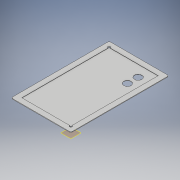
# Autodesk Inventor part: Lid
Saved by Autodesk Inventor 2019 (Build 230136000, 136)
## iProperties
Created: 2018-10-23
Part Number: Lid
Material: Generic
Document SubType Name: Modeling
Designer: Administrator
Density: 1 g/cm^3
Appearance: Default
Author: Administrator
Autodesk Inventor part; units mm, degrees
ref_plane "YZ Plane" through (0, 0, 0) normal (1, 0, 0) x (0, 1, 0)
ref_plane "XZ Plane" through (0, 0, 0) normal (0, 1, 0) x (-1, 0, 0)
ref_plane "XY Plane" through (0, 0, 0) normal (0, 0, 1) x (1, 0, 0)
ref_plane "Work Plane1" through (0, 41.656, 0) normal (0, 1, 0) x (1, 0, 0)
sketch "Sketch2" plane through (0, 41.656, 0) normal (0, 1, 0) x (1, 0, 0)
  line L0 (-118.364, 207.264) -> (-10.414, 207.264) projected
  arc A0 (-4.064, 200.914) -> (-10.414, 207.264) centre (-10.414, 200.914) ccw projected
  line L1 (-4.064, 200.914) -> (-4.064, 10.414) projected
  arc A1 (-10.414, 4.064) -> (-4.064, 10.414) centre (-10.414, 10.414) ccw projected
  line L2 (-10.414, 4.064) -> (-118.364, 4.064) projected
  arc A2 (-124.714, 10.414) -> (-118.364, 4.064) centre (-118.364, 10.414) ccw projected
  line L3 (-124.714, 10.414) -> (-124.714, 200.914) projected
  arc A3 (-118.364, 207.264) -> (-124.714, 200.914) centre (-118.364, 200.914) ccw projected
  line L4 (-128.778, 208.153) -> (-128.778, 3.175) projected
  arc A4 (-128.778, 3.175) -> (-125.603, 0) centre (-125.603, 3.175) ccw projected
  line L5 (-125.603, 0) -> (-3.175, 0) projected
  arc A5 (-3.175, 0) -> (0, 3.175) centre (-3.175, 3.175) ccw projected
  line L6 (0, 3.175) -> (0, 208.153) projected
  arc A6 (0, 208.153) -> (-3.175, 211.328) centre (-3.175, 208.153) ccw projected
  line L7 (-3.175, 211.328) -> (-125.603, 211.328) projected
  arc A7 (-125.603, 211.328) -> (-128.778, 208.153) centre (-125.603, 208.153) ccw projected
  circle A8 centre (-117.348, 199.898) radius 2.794 projected
  circle A9 centre (-11.43, 11.43) radius 2.794 projected
  line L8 (-117.348, 199.898) -> (-11.43, 199.898)
  line L9 (-11.43, 199.898) -> (-11.43, 11.43)
  line L10 (-11.43, 11.43) -> (-117.348, 11.43)
  line L11 (-117.348, 11.43) -> (-117.348, 199.898)
  point P0 (0, 0)
  constraints: 8 end point, 2 parallel, 1 horizontal, 1 perpendicular
extrude "Extrusion5" add sketch "Sketch2" along normal blind 1.27 contours L0 A0 L1 A1 L2 A2 L3 A3 | A7 L7 A6 L6 A5 L5 A4 L4
extrude "Extrusion6" add sketch "Sketch2" along normal blind 0.508 contours L8 L9 A9 L10 L11 A8 | A8 L11 L8 | L9 L10 A9 picked at (-115.5087, 199.6908) picked at (-13.2693, 11.6372)
sketch "Sketch3" plane through (0, 42.164, 0) normal (0, 1, 0) x (1, 0, 0)
  line L0 (-14.224, 11.43) -> (-117.348, 11.43) projected
  line L1 (-114.554, 199.898) -> (-11.43, 199.898) projected
  line L2 (-117.348, 11.43) -> (-62.992, 11.43)
  line L3 (-62.992, 11.43) -> (-62.992, 199.898)
  line L4 (-62.992, 199.898) -> (-117.348, 199.898)
  line L5 (-117.348, 199.898) -> (-117.348, 11.43)
  line L6 (-11.43, 199.898) -> (-62.992, 199.898)
  line L7 (-62.992, 199.898) -> (-62.992, 105.664)
  line L8 (-62.992, 105.664) -> (-11.43, 105.664)
  line L9 (-11.43, 105.664) -> (-11.43, 199.898)
  line L10 (-37.211, 105.664) -> (-62.992, 105.664)
  line L11 (-62.992, 105.664) -> (-62.992, 199.898)
  line L12 (-62.992, 199.898) -> (-37.211, 199.898)
  line L13 (-37.211, 199.898) -> (-37.211, 105.664)
  line L14 (-11.43, 199.898) -> (-11.43, 14.224) projected
  line L15 (-11.43, 199.898) -> (-37.211, 199.898)
  line L16 (-37.211, 199.898) -> (-37.211, 152.781)
  line L17 (-37.211, 152.781) -> (-11.43, 152.781)
  line L18 (-11.43, 152.781) -> (-11.43, 199.898)
  line L19 (-11.43, 105.664) -> (-24.3205, 105.664)
  line L20 (-24.3205, 105.664) -> (-24.3205, 199.898)
  line L21 (-24.3205, 199.898) -> (-11.43, 199.898)
  line L22 (-11.43, 199.898) -> (-11.43, 105.664)
  line L23 (-37.211, 176.3395) -> (-24.3205, 176.3395)
  line L24 (-24.3205, 176.3395) -> (-24.3205, 152.781)
  line L25 (-24.3205, 152.781) -> (-37.211, 152.781)
  line L26 (-37.211, 152.781) -> (-37.211, 176.3395)
  line L27 (-37.211, 105.664) -> (-24.3205, 105.664)
  line L28 (-24.3205, 105.664) -> (-24.3205, 152.781)
  line L29 (-24.3205, 152.781) -> (-37.211, 152.781)
  line L30 (-37.211, 152.781) -> (-37.211, 105.664)
  line L31 (-37.211, 129.2225) -> (-24.3205, 129.2225)
  line L32 (-24.3205, 129.2225) -> (-24.3205, 152.781)
  line L33 (-24.3205, 152.781) -> (-37.211, 152.781)
  line L34 (-37.211, 152.781) -> (-37.211, 129.2225)
  line L35 (-24.3205, 105.664) -> (-30.7657, 105.664)
  line L36 (-30.7657, 105.664) -> (-30.7657, 129.2225)
  line L37 (-30.7657, 129.2225) -> (-24.3205, 129.2225)
  line L38 (-24.3205, 129.2225) -> (-24.3205, 105.664)
  line L39 (-30.7657, 129.2225) -> (-24.3205, 129.2225)
  line L40 (-24.3205, 129.2225) -> (-24.3205, 199.898)
  line L41 (-24.3205, 199.898) -> (-30.7657, 199.898)
  line L42 (-30.7657, 199.898) -> (-30.7657, 129.2225)
  point P0 (0, 0)
  constraints: 80 end point, 20 parallel, 10 horizontal, 10 perpendicular, 9 midpoint
sketch "Sketch4" plane through (0, 42.164, 0) normal (0, 1, 0) x (1, 0, 0)
  point P0 (0, 0)
  point P1 (-30.9206, 152.9754)
  point P2 (-30.9206, 176.1357)
hole "Hole1" at (-30.9206, 42.164, -152.9754) at (-30.9206, 42.164, -176.1357) direction (0, -1, 0) diameter 16.002 depth 8.001 tip angle 118
sketch "Sketch5" plane through (0, 42.164, 0) normal (0, 1, 0) x (1, 0, 0)
  circle A0 centre (-30.9206, 152.9754) radius 8.001 projected
  circle A1 centre (-30.9206, 176.1357) radius 8.001 projected
  line L0 (-30.9206, 152.9754) -> (-38.9216, 152.9754)
  line L1 (-30.9206, 152.9754) -> (-22.9196, 152.9754)
  circle A2 centre (-30.9206, 176.1357) radius 8.001 projected
  line L2 (-38.9216, 176.1357) -> (-30.9206, 176.1357)
  line L3 (-30.9206, 176.1357) -> (-22.9196, 176.1357)
  circle A3 centre (-30.9206, 152.9754) radius 7.5057
  circle A4 centre (-30.9206, 176.1357) radius 7.5057
  line L4 (-30.9206, 152.9754) -> (-38.9216, 152.9754)
  line L5 (-38.9216, 152.9754) -> (-38.9216, 160.4811)
  line L6 (-38.9216, 160.4811) -> (-30.9206, 160.4811)
  line L7 (-30.9206, 160.4811) -> (-30.9206, 152.9754)
  line L8 (-30.9206, 152.9754) -> (-22.9196, 152.9754)
  line L9 (-22.9196, 152.9754) -> (-22.9196, 145.4697)
  line L10 (-22.9196, 145.4697) -> (-30.9206, 145.4697)
  line L11 (-30.9206, 145.4697) -> (-30.9206, 152.9754)
  line L12 (-22.9196, 145.4697) -> (-38.9216, 145.4697)
  line L13 (-38.9216, 145.4697) -> (-38.9216, 160.4811)
  line L14 (-38.9216, 160.4811) -> (-22.9196, 160.4811)
  line L15 (-22.9196, 160.4811) -> (-22.9196, 145.4697)
  line L16 (-30.9206, 176.1357) -> (-22.9196, 176.1357)
  line L17 (-22.9196, 176.1357) -> (-22.9196, 168.63)
  line L18 (-22.9196, 168.63) -> (-30.9206, 168.63)
  line L19 (-30.9206, 168.63) -> (-30.9206, 176.1357)
  line L20 (-30.9206, 176.1357) -> (-38.9216, 176.1357)
  line L21 (-38.9216, 176.1357) -> (-38.9216, 183.6414)
  line L22 (-38.9216, 183.6414) -> (-30.9206, 183.6414)
  line L23 (-30.9206, 183.6414) -> (-30.9206, 176.1357)
  line L24 (-38.9216, 183.6414) -> (-22.9196, 183.6414)
  line L25 (-22.9196, 183.6414) -> (-22.9196, 168.63)
  line L26 (-22.9196, 168.63) -> (-38.9216, 168.63)
  line L27 (-38.9216, 168.63) -> (-38.9216, 183.6414)
  circle A5 centre (-30.9206, 152.9754) radius 8.001
  circle A6 centre (-30.9206, 176.1357) radius 8.001
  line L28 (-33.692, 183.6414) -> (-28.1492, 183.6414)
  arc A7 (-28.1492, 183.6414) -> (-33.692, 183.6414) centre (-30.9206, 176.1357) ccw
  arc A8 (-33.692, 168.63) -> (-28.1492, 168.63) centre (-30.9206, 176.1357) ccw
  line L29 (-33.692, 168.63) -> (-28.1492, 168.63)
  arc A9 (-28.1492, 160.4811) -> (-33.692, 160.4811) centre (-30.9206, 152.9754) ccw
  arc A10 (-33.692, 145.4697) -> (-28.1492, 145.4697) centre (-30.9206, 152.9754) ccw
  line L30 (-33.692, 145.4697) -> (-28.1492, 145.4697)
  line L31 (-33.692, 160.4811) -> (-28.1492, 160.4811)
  point P0 (0, 0)
  dimension "d51" = 15.0114
  dimension "d52" = 15.0114
  dimension "d53" = 15.0114
  dimension "d54" = 15.0114
  dimension "d55" = 16.002
  dimension "d56" = 8.001
  dimension "d57" = 7.5057
  dimension "d58" = 7.5057
  constraints: 64 end point, 20 point on circle, 14 parallel, 12 point on line, 8 centre point, 7 horizontal, 6 concentric, 6 perpendicular, 4 coincident, 2 collinear
  measures "d51" diameter of A3
  measures "d52" diameter of A4
  measures "d53" distance between parallel lines of L6 L12
  measures "d54" distance between parallel lines of L22 L26
  measures "d55" distance between parallel lines of L25 L27
  measures "d56" distance between parallel lines of L11 L15
  measures "d57" distance between parallel lines of L0 L12
  measures "d58" distance between parallel lines of L2 L26
extrude "Extrusion7" add sketch "Sketch5" against normal blind 0.508 contours L14 L6 A0 | A0 L12 L10 | L24 L22 A1 | A1 L26 L18
body "Solid1"
